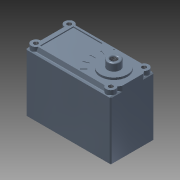
# Autodesk Inventor part: 42
Saved by Autodesk Inventor 2013 (Build 170138000, 138)
## iProperties
Created: 2013-12-28
Material: SAN プラスチック
Document SubType Name: Modeling
Designer: andou
Density: 1.35846 g/cm^3
Mass: 35 g
Surface Area: 65.5794 cm^2
Volume: 25.7645 cm^3
Part Number: 42
Description: 市販品
Author: andou
Title: KRS-2542HV
Autodesk Inventor part; units mm, degrees
note: some values were not read from the file. Chosen so that the rebuilt part matches the saved one: pattern direction of "円形状パターン1"; pattern direction of "円形状パターン2".
ref_plane "YZ Plane" through (0, 0, 0) normal (1, 0, 0) x (0, 1, 0)
ref_plane "XZ Plane" through (0, 0, 0) normal (0, 1, 0) x (-1, 0, 0)
ref_plane "XY Plane" through (0, 0, 0) normal (0, 0, 1) x (1, 0, 0)
sketch "スケッチ1" plane through (0, 0, 0) normal (0, 0, 1) x (1, 0, 0)
  line L0 (-20.5, 10.5) -> (20.5, 10.5)
  line L1 (20.5, 10.5) -> (20.5, -10.5)
  line L2 (20.5, -10.5) -> (-20.5, -10.5)
  line L3 (-20.5, -10.5) -> (-20.5, 10.5)
  point P0 (0, 0)
  dimension "d0" = 21
  dimension "d1" = 10.5
  dimension "d2" = 41
  dimension "d3" = 20.5
  constraints: 8 end point, 2 parallel, 1 horizontal, 1 perpendicular
  measures "d0" distance of L2.end L0.start
  measures "d1" distance from line of L2 point (0, 0)
  measures "d2" distance between parallel lines of L1 L3
  measures "d3" distance from line of L3 point (0, 0)
extrude "押し出し1" add sketch "スケッチ1" along normal blind 30.5
sketch "スケッチ2" plane through (0, 0, 30.5) normal (0, 0, 1) x (1, 0, 0)
  line L0 (20.5, 10.5) -> (20.5, -10.5) projected
  line L1 (-20.5, -10.5) -> (-20.5, 10.5) projected
  line L2 (20.5, -10.5) -> (-20.5, -10.5) projected
  circle A0 centre (-18, 8) radius 1
  circle A1 centre (-18, -8) radius 1
  circle A2 centre (18, 8) radius 1
  circle A3 centre (18, -8) radius 1
  point P0 (0, 0)
  dimension "d6" = 2
  dimension "d7" = 36
  dimension "d8" = 36
  dimension "d9" = 16
  dimension "d10" = 16
  dimension "d11" = 2.5
  dimension "d12" = 2.5
  dimension "d13" = 2.5
  dimension "d14" = 2.5
  constraints: 4 centre point, 3 equal radius
  measures "d6" diameter of A0
  measures "d7" distance of A2.centre A0.centre
  measures "d8" distance of A1.centre A3.centre
  measures "d9" distance of A2.centre A3.centre
  measures "d10" distance of A0.centre A1.centre
  measures "d11" distance from line of L2 A1.centre
  measures "d12" distance from line of L1 A1.centre
  measures "d13" distance from line of A3.centre L2
  measures "d14" distance from line of L0 A2.centre
hole "穴1" at (-18, -8, 30.5) at (-18, 8, 30.5) at (18, -8, 30.5) at (18, 8, 30.5) direction (0, 0, -1) diameter 2 end through all
sketch "スケッチ3" plane through (0, 0, 30.5) normal (0, 0, 1) x (1, 0, 0)
  line L0 (-20.5, 10.5) -> (20.5, 10.5) projected
  circle A0 centre (11.5, 0) radius 6.5
  point P0 (0, 0)
  dimension "d22" = 13
  dimension "d23" = 11.5
  dimension "d24" = 10.5
  constraints: 1 centre point
  measures "d22" diameter of A0
  measures "d23" distance of point (0, 0) A0.centre
  measures "d24" distance from line of L0 A0.centre
extrude "押し出し2" add sketch "スケッチ3" along normal blind 1
sketch "スケッチ4" plane through (11.5, 0, 31.5) normal (0, 0, 1) x (1, 0, 0)
  circle A0 centre (0, 0) radius 6.5 projected
  circle A1 centre (0, 0) radius 3
  point P0 (-11.5, 0)
  dimension "d27" = 6
  constraints: 1 centre point, 1 coincident
  measures "d27" diameter of A1
extrude "押し出し3" add sketch "スケッチ4" along normal blind 3.5 contours A1
sketch "スケッチ5" plane through (11.5, 0, 35) normal (0, 0, 1) x (1, 0, 0)
  circle A0 centre (0, 0) radius 3 projected
  circle A1 centre (0, 0) radius 1.5
  point P0 (-11.5, 0)
  dimension "d30" = 3
  constraints: 1 centre point, 1 coincident
  measures "d30" diameter of A1
hole "穴2" at (11.5, 0, 35) direction (0, 0, -1) diameter 3 depth 8 tip angle 118
sketch "スケッチ6" plane through (0, 0, 30.5) normal (0, 0, 1) x (1, 0, 0)
  line L0 (-20.5, -10.5) -> (-20.5, 10.5) projected
  line L1 (0, 0.25) -> (2.5, 0.25)
  line L2 (2.5, 0.25) -> (2.5, -0.25)
  line L3 (2.5, -0.25) -> (0, -0.25)
  line L4 (0, -0.25) -> (0, 0.25)
  point P0 (0, 0)
  dimension "d38" = 0.5
  dimension "d39" = 0.25
  dimension "d40" = 2.5
  dimension "d41" = 20.5
  constraints: 8 end point, 2 parallel, 1 horizontal, 1 perpendicular
  measures "d38" distance between parallel lines of L1 L3
  measures "d39" distance from line of point (0, 0) L3
  measures "d40" distance between parallel lines of L2 L4
  measures "d41" distance between parallel lines of L0 L4
extrude "押し出し4" cut sketch "スケッチ6" against normal blind 0.25
pattern_circular "円形状パターン1" count 5 over 90 about axis through (11.5, 0, 31) along (0, 0, -1) of "押し出し4" both ways yes
sketch "スケッチ8" plane through (0, 0, 30.5) normal (0, 0, 1) x (1, 0, 0)
  circle A0 centre (11.5, 0) radius 6.5 projected
  circle A1 centre (18, 8) radius 1 projected
  circle A2 centre (18, -8) radius 1 projected
  circle A3 centre (-18, 8) radius 1 projected
  circle A4 centre (-18, -8) radius 1 projected
  line L0 (20.5, 10.5) -> (20.5, -10.5) projected
  line L1 (-20.5, 10.5) -> (20.5, 10.5) projected
  line L2 (-20.5, -10.5) -> (-20.5, 10.5) projected
  line L3 (20.5, -10.5) -> (-20.5, -10.5) projected
  arc A5 (-16.3229, 9.5) -> (-18.5, 5.8063) centre (-18, 8) ccw
  arc A6 (-18.5, -5.8063) -> (-16.3229, -9.5) centre (-18, -8) ccw
  arc A7 (16.3229, -9.5) -> (19.581, -6.3991) centre (18, -8) ccw
  arc A8 (19.581, 6.3991) -> (16.3229, 9.5) centre (18, 8) ccw
  line L4 (-18.5, 5.8063) -> (-18.5, -5.8063)
  line L5 (-16.3229, 9.5) -> (16.3229, 9.5)
  line L6 (-16.3229, -9.5) -> (16.3229, -9.5)
  arc A9 (20.5, 5.0249) -> (19.581, 6.3991) centre (11.5, 0) ccw
  arc A10 (19.581, -6.3991) -> (20.5, -5.0249) centre (11.5, 0) ccw
  point P0 (0, 0)
  dimension "d49" = 4.5
  dimension "d50" = 1
  dimension "d51" = 2
  dimension "d52" = 1
  dimension "d53" = 10.3078
  dimension "d56" = 10.3078
  constraints: 12 point on circle, 6 centre point, 6 end point, 5 coincident, 3 equal radius, 2 perpendicular, 2 point on line, 1 parallel
  measures "d49" diameter of A5
  measures "d50" distance between parallel lines of L1 L5
  measures "d51" distance between parallel lines of L2 L4
  measures "d52" distance between parallel lines of L3 L6
  measures "d53" radius of A9
  measures "d56" radius of A10
extrude "押し出し5" cut sketch "スケッチ8" against normal blind 2 contours L0 A9 A8 L5 A5 L4 A6 L6 A7 A10 L3 L2 L1
chamfer "面取り1" distance 2 angle 15 1 edges at (0, -9.5, 30.5) measured on face at (5.441, -9.5, 29.8333)
chamfer "面取り2" distance 2 angle 15 1 edges at (-18.5, 0, 30.5) measured on face at (-18.5, -1.9354, 29.8333)
chamfer "面取り3" distance 2 angle 15 1 edges at (0, 9.5, 30.5) measured on face at (-5.441, 9.5, 29.8333)
sketch "スケッチ10" plane through (0, 0, 30.5) normal (0, 0, 1) x (1, 0, 0)
  line L0 (-16, 8) -> (-2, 8)
  line L1 (-2, 8) -> (-2, -8)
  line L2 (-2, -8) -> (-16, -8)
  line L3 (-16, -8) -> (-16, 8)
  point P0 (0, 0)
  dimension "d69" = 16
  dimension "d70" = 14
  dimension "d72" = 2
  dimension "d73" = 8
  constraints: 8 end point, 2 parallel, 1 horizontal, 1 perpendicular
  measures "d69" distance between parallel lines of L0 L2
  measures "d70" distance of L1.end L2.end
  measures "d72" distance from line of point (0, 0) L1
  measures "d73" distance from line of point (0, 0) L2
extrude "押し出し6" cut sketch "スケッチ10" against normal blind 0.5
sketch "スケッチ12" plane through (0, 0, 0) normal (0, 0, -1) x (-1, 0, 0)
  circle A0 centre (-18, 8) radius 1 projected
  circle A1 centre (-18, -8) radius 1 projected
  circle A2 centre (18, 8) radius 1 projected
  circle A3 centre (18, -8) radius 1 projected
  circle A4 centre (-18, 8) radius 2.25
  circle A5 centre (-18, -8) radius 2.25
  circle A6 centre (18, -8) radius 2.25
  circle A7 centre (18, 8) radius 2.25
  point P0 (0, 0)
  dimension "d76" = 4.5
  constraints: 4 centre point, 4 coincident, 3 equal radius
  measures "d76" diameter of A4
hole "穴3" at (-18, 8, 0) at (-18, -8, 0) at (18, -8, 0) at (18, 8, 0) direction (0, 0, 1) diameter 4 depth 2
sketch "スケッチ13" plane through (0, 0, 0) normal (0, 0, -1) x (-1, 0, 0)
  line L0 (20.5, 10.5) -> (-20.5, 10.5) projected
  circle A0 centre (-11.5, 0) radius 6.5
  point P0 (0, 0)
  dimension "d84" = 13
  dimension "d85" = 11.5
  dimension "d86" = 10.5
  constraints: 1 centre point
  measures "d84" diameter of A0
  measures "d85" distance of point (0, 0) A0.centre
  measures "d86" distance from line of L0 A0.centre
extrude "押し出し7" add sketch "スケッチ13" along normal blind 1
sketch "スケッチ14" plane through (11.5, 0, -1) normal (0, 0, -1) x (-1, 0, 0)
  circle A0 centre (0, 0) radius 6.5 projected
  circle A1 centre (0, 0) radius 3.5
  point P0 (11.5, 0)
  dimension "d89" = 7
  constraints: 1 centre point, 1 coincident
  measures "d89" diameter of A1
extrude "押し出し8" add sketch "スケッチ14" along normal blind 2 contours A1
sketch "スケッチ15" plane through (11.5, 0, -3) normal (0, 0, -1) x (-1, 0, 0)
  circle A0 centre (0, 0) radius 3.5 projected
  circle A1 centre (0, 0) radius 1.5
  point P0 (11.5, 0)
  dimension "d92" = 3
  constraints: 1 centre point, 1 coincident
  measures "d92" diameter of A1
hole "穴4" at (11.5, 0, -3) direction (0, 0, 1) diameter 3 depth 6 tip angle 118
sketch "スケッチ16" plane through (0, 0, 0) normal (0, 0, -1) x (-1, 0, 0)
  line L0 (20.5, -10.5) -> (20.5, 10.5) projected
  line L1 (-4.5, 0.25) -> (-2, 0.25)
  line L2 (-2, 0.25) -> (-2, -0.25)
  line L3 (-2, -0.25) -> (-4.5, -0.25)
  line L4 (-4.5, -0.25) -> (-4.5, 0.25)
  point P0 (0, 0)
  dimension "d100" = 2.5
  dimension "d101" = 0.25
  dimension "d102" = 0.5
  dimension "d103" = 22.5
  constraints: 8 end point, 2 parallel, 1 horizontal, 1 perpendicular
  measures "d100" distance of L2.end L3.end
  measures "d101" distance from line of point (0, 0) L3
  measures "d102" distance of L1.end L2.end
  measures "d103" distance between parallel lines of L0 L2
extrude "押し出し9" cut sketch "スケッチ16" against normal blind 0.25
pattern_circular "円形状パターン2" count 9 over 180 about axis through (11.5, 0, 0) along (0, 0, -1) of "押し出し9" both ways yes
sketch "スケッチ18" plane through (0, 0, 0) normal (0, 0, -1) x (-1, 0, 0)
  line L0 (0.5, 2.5) -> (6.5, 2.5)
  line L1 (6.5, 2.5) -> (6.5, 6)
  line L2 (6.5, 6) -> (0.5, 6)
  line L3 (0.5, 6) -> (0.5, 2.5)
  line L4 (0.5, -2.5) -> (6.5, -2.5)
  line L5 (6.5, -2.5) -> (6.5, -6)
  line L6 (6.5, -6) -> (0.5, -6)
  line L7 (0.5, -6) -> (0.5, -2.5)
  point P0 (0, 0)
  dimension "d109" = 2.5
  dimension "d110" = 2.5
  dimension "d111" = 6
  dimension "d112" = 3.5
  dimension "d113" = 0.5
  dimension "d114" = 0.5
  constraints: 16 end point, 4 parallel, 2 equal length, 2 horizontal, 2 perpendicular
  measures "d109" distance from line of point (0, 0) L0
  measures "d110" distance from line of point (0, 0) L4
  measures "d111" distance of L5.end L6.end
  measures "d112" distance of L4.end L5.end
  measures "d113" distance from line of point (0, 0) L3
  measures "d114" distance from line of point (0, 0) L7
extrude "押し出し10" add sketch "スケッチ18" along normal blind 1
chamfer "面取り5" distance 0.5 angle 45 14 edges at (-20.5, 0, 0) (0, -10.5, 0) (0, 10.5, 0) (20.5, 0, 0) (0, -10.5, 28.5) (-20.5, 0, 28.5) (0, 10.5, 28.5) (20.5, 7.7625, 28.5) (20.5, -7.7625, 28.5) (-20.5, -10.5, 14.25) (20.5, -10.5, 14.25) (20.5, 10.5, 14.25) (-20.5, 10.5, 14.25) (15, 0, -3)
fillet "フィレット2" radius 0.5 2 edges at (8.5, 0, 35) (11.5, 1.5, 35)
thread "ねじ1" size "M3x0.5" class "6H" standard "ANSI Metric M Profile" full length
thread "ねじ2" size "M2x0.4" class "6H" standard "ANSI Metric M Profile" full length
thread "ねじ3" size "M2x0.4" class "6H" standard "ANSI Metric M Profile" full length
thread "ねじ4" size "M2x0.4" class "6H" standard "ANSI Metric M Profile" full length
thread "ねじ5" size "M2x0.4" class "6H" standard "ANSI Metric M Profile" full length
sketch "スケッチ19" plane through (11.5, 0, 35) normal (0, 0, 1) x (1, 0, 0)
  circle A0 centre (0, 0) radius 2.5 projected
  circle A1 centre (2.25, 0) radius 0.25
  point P0 (-11.5, 0)
  dimension "d135" = 0.5
  dimension "d136" = 2.25
  constraints: 1 centre point
  measures "d135" diameter of A1
  measures "d136" distance of A0.centre A1.centre
hole "穴5" at (13.75, 0, 35) direction (0, 0, -1) diameter 0.5 depth 0.1
